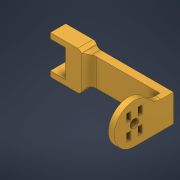
# Autodesk Inventor part: Roll Pitch Axis Support
Saved by Autodesk Inventor 2022 (Build 260153000, 153)
## iProperties
Created: 2021-07-30
Part Number: Roll Pitch Axis Support
Material: Generic
Document SubType Name: Modeling
Designer: sidsa
Density: 1 g/cm^3
Appearance: Brass - Satin
Author: sidsa
Autodesk Inventor part; units mm, degrees
ref_plane "YZ Plane" through (0, 0, 0) normal (1, 0, 0) x (0, 1, 0)
ref_plane "XZ Plane" through (0, 0, 0) normal (0, 1, 0) x (-1, 0, 0)
ref_plane "XY Plane" through (0, 0, 0) normal (0, 0, 1) x (1, 0, 0)
sketch "Sketch1" plane through (0, 0, 0) normal (0, 0, 1) x (1, 0, 0)
  line L0 (0, 0) -> (25.4, 0)
  line L1 (25.4, 0) -> (25.4, 31.75)
  line L2 (25.4, 31.75) -> (0, 31.75)
  line L3 (0, 31.75) -> (0, 0)
  line L4 (0, 15.875) -> (25.4, 15.875)
  line L5 (12.4968, 4.4958) -> (0, 4.4958)
  line L6 (0, 4.4958) -> (0, 27.2542)
  line L7 (0, 27.2542) -> (12.4968, 27.2542)
  line L8 (12.4968, 27.2542) -> (12.4968, 4.4958)
  line L9 (12.4968, 4.4958) -> (0, 27.2542) construction
  line L10 (0, 4.4958) -> (12.4968, 27.2542) construction
  line L11 (25.4, 4.4958) -> (25.4, 27.2542)
  line L12 (25.4, 27.2542) -> (88.9, 27.2542)
  line L13 (88.9, 27.2542) -> (88.9, 4.4958)
  line L14 (88.9, 4.4958) -> (25.4, 4.4958)
  point P0 (6.2484, 15.875)
  point P1 (0, 4.4958)
  dimension "d0" = 25.4
  dimension "d1" = 31.75
  dimension "d2" = 22.7584
  dimension "d3" = 12.4968
  dimension "d4" = 63.5
  constraints: 30 end point, 6 parallel, 4 midpoint, 4 point on line, 3 perpendicular, 2 collinear, 2 horizontal
  measures "d0" distance of L2.end L1.end
  measures "d1" distance of L0.end L1.end
  measures "d2" distance of L7.end L5.start
  measures "d3" distance of L6.end L7.end
  measures "d4" distance of L11.end L12.end
extrude "Extrusion1" add sketch "Sketch1" along normal blind 6.35 contours L3 L5 L8 L4 L1 L0 | L1 L12 L13 L14 | L4 L8 L7 L3 L2 L1
fillet "Fillet1" radius 3.175 4 edges at (25.4, 27.2542, 3.175) (25.4, 31.75, 3.175) (25.4, 4.4958, 3.175) (25.4, 0, 3.175)
sketch "Sketch4" plane through (0, 0, 6.35) normal (0, 0, 1) x (1, 0, 0)
  arc A0 (22.5017, 0) -> (25.5384, 2.2479) centre (22.5017, 3.175) ccw projected
  arc A1 (28.575, 4.4958) -> (25.5384, 2.2479) centre (28.575, 1.3208) ccw projected
  line L0 (28.575, 4.4958) -> (88.9, 4.4958) projected
  line L1 (88.9, 4.4958) -> (88.9, 27.2542) projected
  line L2 (88.9, 27.2542) -> (28.575, 27.2542) projected
  arc A2 (25.5384, 29.5021) -> (28.575, 27.2542) centre (28.575, 30.4292) ccw projected
  arc A3 (25.5384, 29.5021) -> (22.5017, 31.75) centre (22.5017, 28.575) ccw projected
  line L3 (22.5017, 31.75) -> (0, 31.75) projected
  line L4 (0, 31.75) -> (0, 27.2542) projected
  line L5 (0, 27.2542) -> (12.4968, 27.2542) projected
  line L6 (12.4968, 27.2542) -> (12.4968, 4.4958) projected
  line L7 (12.4968, 4.4958) -> (0, 4.4958) projected
  line L8 (0, 4.4958) -> (0, 0) projected
  line L9 (0, 0) -> (22.5017, 0) projected
  arc A4 (25.5384, 29.5021) -> (28.575, 27.2542) centre (28.575, 30.4292) ccw projected
  arc A5 (28.575, 4.4958) -> (25.5384, 2.2479) centre (28.575, 1.3208) ccw projected
  line L10 (25.5384, 29.5021) -> (25.5384, 2.2479)
  constraints: 2 end point, 1 vertical
extrude "Extrusion4" add sketch "Sketch4" along normal blind 6.35 contours L9 L8 L7 L6 L5 L4 L3 A3 L10 A0
fillet "Fillet4" radius 6.35 1 edges at (25.5384, 15.875, 6.35)
sketch "Sketch5" plane through (88.9, 4.4958, 0) normal (1, 0, 0) x (0, 0, -1)
  line L0 (0, 22.7584) -> (0, 0) projected
  line L1 (0, 0) -> (-32.4104, 0)
  circle A0 centre (-32.4104, 16.51) radius 16.51
  line L2 (-7.283, 22.7584) -> (0, 22.7584) projected
  line L3 (-6.3347, 22.7584) -> (-17.1285, 22.7584)
  circle A1 centre (-32.4104, 16.51) radius 3.4925
  point P0 (0, -4.4958)
  dimension "d17" = 32.4104
  dimension "d18" = 33.02
  dimension "d19" = 6.985
  constraints: 4 end point, 2 centre point, 2 point on circle, 1 coincident, 1 collinear, 1 horizontal, 1 point on line
  measures "d17" distance of L0.end L1.end
  measures "d18" diameter of A0
  measures "d19" diameter of A1
extrude "Extrusion5" add sketch "Sketch5" against normal blind 4.7625
fillet "Fillet5" radius 12.7 1 edges at (86.5188, 27.2542, 17.1285)
sketch "Sketch6" plane through (88.9, 4.4958, 0) normal (1, 0, 0) x (0, 0, -1)
  circle A0 centre (-32.4104, 16.51) radius 3.4925 projected
  line L0 (0, 0) -> (0, 22.7584) projected
  line L1 (0, 22.7584) -> (-10.1802, 22.7584) projected
  arc A1 (-19.8455, 27.22) -> (-10.1802, 22.7584) centre (-10.1802, 35.4584) ccw projected
  arc A2 (-19.8455, 27.22) -> (-32.4104, 0) centre (-32.4104, 16.51) ccw projected
  line L2 (0, 0) -> (-32.4104, 0) projected
  arc A3 (-19.8455, 27.22) -> (-32.4104, 0) centre (-32.4104, 16.51) ccw projected
  line L3 (-32.4104, 16.51) -> (-48.9204, 16.51)
  line L4 (-32.4104, 16.51) -> (-32.4104, 33.02)
  line L5 (-35.5854, 20.32) -> (-38.7604, 20.32)
  line L6 (-38.7604, 20.32) -> (-38.7604, 26.67)
  line L7 (-38.7604, 26.67) -> (-35.5854, 26.67)
  line L8 (-35.5854, 26.67) -> (-35.5854, 20.32)
  line L9 (-32.4104, 16.51) -> (-15.9004, 16.51)
  line L10 (-29.2354, 20.32) -> (-26.0604, 20.32)
  line L11 (-26.0604, 20.32) -> (-26.0604, 26.67)
  line L12 (-26.0604, 26.67) -> (-29.2354, 26.67)
  line L13 (-29.2354, 26.67) -> (-29.2354, 20.32)
  line L14 (-35.5854, 12.7) -> (-38.7604, 12.7)
  line L15 (-38.7604, 12.7) -> (-38.7604, 6.35)
  line L16 (-38.7604, 6.35) -> (-35.5854, 6.35)
  line L17 (-35.5854, 6.35) -> (-35.5854, 12.7)
  line L18 (-29.2354, 6.35) -> (-29.2354, 12.7)
  line L19 (-29.2354, 12.7) -> (-26.0604, 12.7)
  line L20 (-26.0604, 12.7) -> (-26.0604, 6.35)
  line L21 (-26.0604, 6.35) -> (-29.2354, 6.35)
  point P0 (0, -4.4958)
  dimension "d23" = 6.35
  dimension "d24" = 6.35
  dimension "d25" = 3.175
  dimension "d26" = 7.62
  constraints: 38 end point, 13 symmetric about line, 2 horizontal, 2 parallel, 2 perpendicular, 2 point on circle
  measures "d23" diameter of L8 L4
  measures "d24" distance of L7.end L5.start
  measures "d25" distance of L5.start L5.end
  measures "d26" diameter of L5 L3
extrude "Extrusion6" cut sketch "Sketch6" against normal blind 4.7625 contours L5 L6 L7 L8 | L13 L12 L11 L10 | L17 L16 L15 L14 | L18 L19 L20 L21
body "Solid1"
